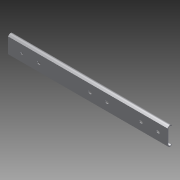
# Autodesk Inventor part: MICHAUD CHAILLY B3 - 21 - 30 - 1
Saved by Autodesk Inventor 2011 SP1 (Build 150282100, 282)
## iProperties
Created: 2012-12-20
Part Number: MICHAUD CHAILLY B3 - 21 - 30 - 1
Catalog Web Link: www.cadenas.de
Description: Modèle B3-21-1-GLISSIERE DOUBLE COURSE 75%
Vendor: EMILEMAURIN
Document SubType Name: Modeling
Designer: PARTuser1
Manufacturer: EMILEMAURIN
Density: 1 g/cm^3
Category: PARTsolutions
Company: EMILEMAURIN
Title: MICHAUD CHAILLY B3 - 21 - 30 - 1
Author: Cadenas PARTsolutions
Comments: GLISSIERE DOUBLE COURSE 75%
PSOL_IDENT_0: {\\10.0.0.242\data_v9\23d-libs\michaud_chailly_transmission\guidage\autres_composants\glissieres_a_b
PSOL_IDENT_1: illes\b3_21\b3_21_1.prj},214 {VTYP=3D},{NB=MICHAUD CHAILLY B3 - 21 - 30 - 1},{LINA=MICHAUD CHAILLY B
PSOL_IDENT_2: 3 - 21 - 30 - 1},{NN=Modèle B3-21-1},{DATE=11.03.2011 14:16:37},{GEOMDATE=10.04.2007 10:37:00},{VERS
PSOL_IDENT_3: ION=},{LINEID=20},{LINESUBID=-1},{WBVAR=}  {NB=michaud_chailly_B3 - 21 - 30_1},{LINA=MICHAUD CHAILLY
PSOL_IDENT_4: B3 - 21 - 30 - 1},{KT=DUMMY},{REF=B3 - 21 - 30},{L=300},{L1=152.900},{L2=184.900},{L3=248.900},{L4=
PSOL_IDENT_5: 280.900}
CNS_NT: GLISSIERE DOUBLE COURSE 75%
CNS_NB: michaud_chailly_B3 - 21 - 30_1
CNS_NBSYN: michaud_chailly_$REF._1
CNS_LINA: MICHAUD CHAILLY B3 - 21 - 30 - 1
CNS_REF: B3 - 21 - 30
CNS_L: 300
CNS_L1: 152.900
CNS_L2: 184.900
CNS_L3: 248.900
CNS_L4: 280.900
SUPPLIER: EMILEMAURIN
ARTICLENO: MICHAUD CHAILLY B3 - 21 - 30 - 1
BOMINFO: MICHAUD CHAILLY B3 - 21 - 30 - 1
CREATOR: CADENAS GmbH
Autodesk Inventor part; units mm, degrees
sketch "Esquisse_1" plane through (0, 0, 0) normal (1, 0, 0) x (0, 1, 0)
  arc A0 (8.5002, 15.4448) -> (1.9449, 16.4446) centre (4.8548, 13.5338) ccw
  line L0 (1.9449, 16.4446) -> (0, 14.5)
  line L1 (0, 14.5) -> (0, -14.5)
  line L2 (0, -14.5) -> (1.9449, -16.4446)
  arc A1 (1.9449, -16.4446) -> (8.5001, -15.4451) centre (4.8548, -13.5338) ccw
  line L3 (8.5001, -15.4451) -> (7.1713, -14.7492)
  arc A2 (3.0052, -15.3838) -> (7.1713, -14.7492) centre (4.8548, -13.5337) ccw
  line L4 (3.0052, -15.3838) -> (1.5, -13.879)
  line L5 (1.5, -13.879) -> (1.5, 13.879)
  line L6 (1.5, 13.879) -> (3.0052, 15.3838)
  arc A3 (7.1713, 14.7492) -> (3.0052, 15.3838) centre (4.8548, 13.5337) ccw
  line L7 (7.1713, 14.7492) -> (8.5002, 15.4448)
  constraints: 16 end point, 8 point on circle, 4 centre point
extrude "Extrusion1" add sketch "Esquisse_1" along normal blind 300
sketch "Sketch2" plane through (0, 0, -14.5) normal (0, -1, 0) x (1, 0, 0)
  point P0 (26, 14.5)
hole "Drilling 1" at (26, 0, 0) direction (0, 1, 0) diameter 4.3 depth 1.5
sketch "Esquisse_3" plane through (0, 0, 0) normal (0, 1, 0) x (-1, 0, 0)
  arc A0 (-56.9, -2.15) -> (-56.9, 2.15) centre (-56.9, 0) ccw
  line L0 (-56.9, 2.15) -> (-59.1, 2.15)
  arc A1 (-59.1, 2.15) -> (-59.1, -2.15) centre (-59.1, 0) ccw
  line L1 (-59.1, -2.15) -> (-56.9, -2.15)
  constraints: 4 end point, 4 point on circle, 2 centre point
extrude "Extrusion2" cut sketch "Esquisse_3" along normal blind 1.5
sketch "Esquisse_4" plane through (0, 0, 0) normal (0, 1, 0) x (-1, 0, 0)
  arc A0 (-152.9, -2.15) -> (-152.9, 2.15) centre (-152.9, 0) ccw
  line L0 (-152.9, 2.15) -> (-155.1, 2.15)
  arc A1 (-155.1, 2.15) -> (-155.1, -2.15) centre (-155.1, 0) ccw
  line L1 (-155.1, -2.15) -> (-152.9, -2.15)
  constraints: 4 end point, 4 point on circle, 2 centre point
extrude "Extrusion3" cut sketch "Esquisse_4" along normal blind 1.5
sketch "Esquisse_5" plane through (0, 0, 0) normal (0, 1, 0) x (-1, 0, 0)
  arc A0 (-184.9, -2.15) -> (-184.9, 2.15) centre (-184.9, 0) ccw
  line L0 (-184.9, 2.15) -> (-187.1, 2.15)
  arc A1 (-187.1, 2.15) -> (-187.1, -2.15) centre (-187.1, 0) ccw
  line L1 (-187.1, -2.15) -> (-184.9, -2.15)
  constraints: 4 end point, 4 point on circle, 2 centre point
extrude "Extrusion4" cut sketch "Esquisse_5" along normal blind 1.5
sketch "Esquisse_6" plane through (0, 0, 0) normal (0, 1, 0) x (-1, 0, 0)
  arc A0 (-248.9, -2.15) -> (-248.9, 2.15) centre (-248.9, 0) ccw
  line L0 (-248.9, 2.15) -> (-251.1, 2.15)
  arc A1 (-251.1, 2.15) -> (-251.1, -2.15) centre (-251.1, 0) ccw
  line L1 (-251.1, -2.15) -> (-248.9, -2.15)
  constraints: 4 end point, 4 point on circle, 2 centre point
extrude "Extrusion5" cut sketch "Esquisse_6" along normal blind 1.5
sketch "Esquisse_7" plane through (0, 0, 0) normal (0, 1, 0) x (-1, 0, 0)
  arc A0 (-280.9, -2.15) -> (-280.9, 2.15) centre (-280.9, 0) ccw
  line L0 (-280.9, 2.15) -> (-283.1, 2.15)
  arc A1 (-283.1, 2.15) -> (-283.1, -2.15) centre (-283.1, 0) ccw
  line L1 (-283.1, -2.15) -> (-280.9, -2.15)
  constraints: 4 end point, 4 point on circle, 2 centre point
extrude "Extrusion6" cut sketch "Esquisse_7" along normal blind 1.5
ref_plane "IP0_XY" through (0, 0, 0) normal (-1, 0, 0) x (0, 0, -1)
ref_plane "IP0_YZ" through (0, 0, 0) normal (0, 0, -1) x (0, -1, 0)
ref_plane "IP0_ZX" through (0, 0, 0) normal (0, -1, 0) x (-1, 0, 0)
ref_plane "IP1_XY" through (2.5, 0, 0) normal (1, 0, 0) x (0, 0, -1)
ref_plane "IP1_YZ" through (2.5, 0, 0) normal (0, 0, -1) x (0, 1, 0)
ref_plane "IP1_ZX" through (2.5, 0, 0) normal (0, 1, 0) x (1, 0, 0)
body "Solid1"
